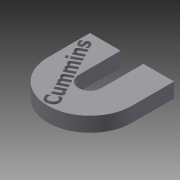
# Autodesk Inventor part: Cummins
Saved by Autodesk Inventor 2015 SP2 (Build 190223200, 223)
## iProperties
Created: 2015-09-30
Part Number: Cummins
Material: Generic
Document SubType Name: Modeling
Designer: KC-019
Density: 1 g/cm^3
Appearance: Default
Author: KC-019
Autodesk Inventor part; units mm, degrees
ref_plane "YZ Plane" through (0, 0, 0) normal (1, 0, 0) x (0, 1, 0)
ref_plane "XZ Plane" through (0, 0, 0) normal (0, 1, 0) x (-1, 0, 0)
ref_plane "XY Plane" through (0, 0, 0) normal (0, 0, 1) x (1, 0, 0)
sketch "Sketch1" plane through (0, 0, 0) normal (0, 1, 0) x (-1, 0, 0)
  line L0 (0, 0) -> (-50.8, 0)
  line L1 (-50.8, 0) -> (-50.8, -25.4)
  line L2 (-50.8, -25.4) -> (0, -25.4)
  line L3 (0, -25.4) -> (0, 0)
  arc A0 (0, 0) -> (-50.8, 0) centre (-25.4, 0) ccw
  line L4 (0, -25.4) -> (-18.5166, -25.4)
  line L5 (-18.5166, -25.4) -> (-32.2834, -25.4)
  line L6 (-32.2834, -25.4) -> (-50.8, -25.4)
  arc A1 (-18.5166, 0) -> (-32.2834, 0) centre (-25.4, 0) ccw
  line L7 (-18.5166, 0) -> (-18.5166, -25.4)
  line L8 (-32.2834, 0) -> (-32.2834, -25.4)
  dimension "d0" = 50.8
  dimension "d1" = 25.4
  dimension "d2" = 18.5166
  dimension "d3" = 13.7668
  dimension "d4" = 18.5166
  constraints: 18 end point, 4 point on circle, 4 point on line, 2 centre point, 2 parallel, 2 perpendicular, 1 coincident, 1 collinear, 1 horizontal, 1 midpoint, 1 tangent
  measures "d0" distance of L2.end L1.end
  measures "d1" distance of L0.end L1.end
  measures "d2" distance of L2.end L4.end
  measures "d3" distance of L4.end L5.end
  measures "d4" distance of L5.end L1.end
extrude "Extrusion1" add sketch "Sketch1" along normal blind 8.89 contours L3 L2 L7 L0 | L0 A1 A0 | L0 L8 L2 L1
sketch "Sketch2" plane through (0, 8.89, 0) normal (0, 1, 0) x (1, 0, 0)
  line L0 (21.5324, -26.082) -> (7.577, 0.2641)
  line L1 (7.577, 0.2641) -> (49.2759, 22.3519)
  line L2 (49.2759, 22.3519) -> (63.2313, -3.9942)
  line L3 (63.2313, -3.9942) -> (21.5324, -26.082)
  spline S0 degree 2 poles (26.8827, -18.5591) (27.6996, -20.1014) (26.7936, -22.8973) (25.1071, -23.7907) knots 0 0 0 1 2 2 2
  spline S1 degree 2 poles (25.1071, -23.7907) (23.4816, -24.6517) (20.5845, -23.8632) (19.7676, -22.3209) knots 0 0 0 1 2 2 2
  spline S2 degree 2 poles (19.7676, -22.3209) (19.553, -21.9159) (19.3006, -21.2113) (19.2196, -20.8706) knots 0 0 0 1 2 2 2
  spline S3 degree 2 poles (19.2196, -20.8706) (19.1683, -20.5994) (19.1159, -19.9238) (19.1136, -19.7048) knots 0 0 0 1 2 2 2
  line L4 (19.1136, -19.7048) -> (20.7446, -18.8409)
  line L5 (20.7446, -18.8409) -> (20.8357, -19.0128)
  spline S4 degree 2 poles (20.8357, -19.0128) (20.7923, -19.1992) (20.6815, -19.741) (20.6636, -20.056) knots 0 0 0 1 2 2 2
  spline S5 degree 2 poles (20.6636, -20.056) (20.6402, -20.3739) (20.7376, -21.054) (20.9051, -21.3702) knots 0 0 0 1 2 2 2
  spline S6 degree 2 poles (20.9051, -21.3702) (21.102, -21.7419) (21.6612, -22.2343) (22.1051, -22.3615) knots 0 0 0 1 2 2 2
  spline S7 degree 2 poles (22.1051, -22.3615) (22.501, -22.4786) (23.5675, -22.3328) (24.1722, -22.0125) knots 0 0 0 1 2 2 2
  spline S8 degree 2 poles (24.1722, -22.0125) (24.8102, -21.6745) (25.502, -20.8748) (25.6213, -20.4563) knots 0 0 0 1 2 2 2
  spline S9 degree 2 poles (25.6213, -20.4563) (25.741, -20.0519) (25.6217, -19.2768) (25.4483, -18.9495) knots 0 0 0 1 2 2 2
  spline S10 degree 2 poles (25.4483, -18.9495) (25.2691, -18.6111) (24.7154, -18.1157) (24.4651, -17.9784) knots 0 0 0 1 2 2 2
  spline S11 degree 2 poles (24.4651, -17.9784) (24.203, -17.8189) (23.7238, -17.6251) (23.5397, -17.5592) knots 0 0 0 1 2 2 2
  line L6 (23.5397, -17.5592) -> (23.4574, -17.4039)
  line L7 (23.4574, -17.4039) -> (25.0663, -16.5517)
  spline S12 degree 2 poles (25.0663, -16.5517) (25.255, -16.6933) (25.7384, -17.0695) (25.9571, -17.2946) knots 0 0 0 1 2 2 2
  spline S13 degree 2 poles (25.9571, -17.2946) (26.2274, -17.5635) (26.6241, -18.0709) (26.8827, -18.5591) knots 0 0 0 1 2 2 2
  line L8 (22.4944, -10.5966) -> (23.3466, -12.2054)
  line L9 (23.3466, -12.2054) -> (22.7752, -12.5081)
  spline S14 degree 2 poles (22.7752, -12.5081) (23.3451, -12.739) (24.0815, -13.2441) (24.3372, -13.7267) knots 0 0 0 1 2 2 2
  spline S15 degree 2 poles (24.3372, -13.7267) (24.7427, -14.4923) (24.2273, -15.8665) (23.2509, -16.3837) knots 0 0 0 1 2 2 2
  line L10 (23.2509, -16.3837) -> (19.889, -18.1645)
  line L11 (19.889, -18.1645) -> (19.0309, -16.5445)
  line L12 (19.0309, -16.5445) -> (21.594, -15.1869)
  spline S16 degree 2 poles (21.594, -15.1869) (21.9934, -14.9753) (22.4833, -14.6661) (22.6141, -14.4974) knots 0 0 0 1 2 2 2
  spline S17 degree 2 poles (22.6141, -14.4974) (22.7338, -14.3345) (22.7386, -13.9412) (22.5917, -13.6638) knots 0 0 0 1 2 2 2
  spline S18 degree 2 poles (22.5917, -13.6638) (22.5036, -13.4974) (22.0903, -13.1195) (21.8432, -13.0018) knots 0 0 0 1 2 2 2
  line L13 (21.8432, -13.0018) -> (18.1817, -14.9412)
  line L14 (18.1817, -14.9412) -> (17.3295, -13.3324)
  line L15 (17.3295, -13.3324) -> (22.4944, -10.5966)
  line L16 (18.5773, -3.2014) -> (15.9976, -4.5679)
  spline S19 degree 2 poles (15.9976, -4.5679) (15.6148, -4.7706) (15.108, -5.0746) (14.9768, -5.2293) knots 0 0 0 1 2 2 2
  spline S20 degree 2 poles (14.9768, -5.2293) (14.8486, -5.3896) (14.8516, -5.7574) (14.9897, -6.0182) knots 0 0 0 1 2 2 2
  spline S21 degree 2 poles (14.9897, -6.0182) (15.0867, -6.2013) (15.4356, -6.4711) (15.6971, -6.6026) knots 0 0 0 1 2 2 2
  line L17 (15.6971, -6.6026) -> (19.353, -4.666)
  line L18 (19.353, -4.666) -> (20.2111, -6.286)
  line L19 (20.2111, -6.286) -> (17.6314, -7.6524)
  spline S22 degree 2 poles (17.6314, -7.6524) (17.2542, -7.8522) (16.7448, -8.1647) (16.6136, -8.3194) knots 0 0 0 1 2 2 2
  spline S23 degree 2 poles (16.6136, -8.3194) (16.4854, -8.4797) (16.4884, -8.8475) (16.6265, -9.1083) knots 0 0 0 1 2 2 2
  spline S24 degree 2 poles (16.6265, -9.1083) (16.7294, -9.3024) (17.1152, -9.5883) (17.3368, -9.6982) knots 0 0 0 1 2 2 2
  line L20 (17.3368, -9.6982) -> (20.9928, -7.7617)
  line L21 (20.9928, -7.7617) -> (21.845, -9.3705)
  line L22 (21.845, -9.3705) -> (16.6801, -12.1063)
  line L23 (16.6801, -12.1063) -> (15.8279, -10.4975)
  line L24 (15.8279, -10.4975) -> (16.3993, -10.1948)
  spline S25 degree 2 poles (16.3993, -10.1948) (15.8578, -9.9773) (15.1073, -9.4725) (14.8752, -9.0343) knots 0 0 0 1 2 2 2
  spline S26 degree 2 poles (14.8752, -9.0343) (14.6254, -8.5627) (14.6927, -7.6035) (15.0422, -7.1768) knots 0 0 0 1 2 2 2
  spline S27 degree 2 poles (15.0422, -7.1768) (14.3656, -6.9456) (13.4646, -6.3713) (13.2413, -5.9497) knots 0 0 0 1 2 2 2
  spline S28 degree 2 poles (13.2413, -5.9497) (13.0503, -5.5891) (12.9751, -4.8972) (13.1052, -4.5796) knots 0 0 0 1 2 2 2
  spline S29 degree 2 poles (13.1052, -4.5796) (13.2403, -4.231) (13.808, -3.6532) (14.3573, -3.3623) knots 0 0 0 1 2 2 2
  line L25 (14.3573, -3.3623) -> (17.7192, -1.5815)
  line L26 (17.7192, -1.5815) -> (18.5773, -3.2014)
  line L27 (13.8226, 5.7748) -> (11.2429, 4.4083)
  spline S30 degree 2 poles (11.2429, 4.4083) (10.8601, 4.2056) (10.3533, 3.9016) (10.2221, 3.7469) knots 0 0 0 1 2 2 2
  spline S31 degree 2 poles (10.2221, 3.7469) (10.0939, 3.5866) (10.0969, 3.2188) (10.235, 2.958) knots 0 0 0 1 2 2 2
  spline S32 degree 2 poles (10.235, 2.958) (10.332, 2.775) (10.681, 2.5051) (10.9424, 2.3737) knots 0 0 0 1 2 2 2
  line L28 (10.9424, 2.3737) -> (14.5984, 4.3102)
  line L29 (14.5984, 4.3102) -> (15.4564, 2.6903)
  line L30 (15.4564, 2.6903) -> (12.8768, 1.3238)
  spline S33 degree 2 poles (12.8768, 1.3238) (12.4995, 1.124) (11.9901, 0.8115) (11.8589, 0.6568) knots 0 0 0 1 2 2 2
  spline S34 degree 2 poles (11.8589, 0.6568) (11.7307, 0.4965) (11.7337, 0.1287) (11.8718, -0.132) knots 0 0 0 1 2 2 2
  spline S35 degree 2 poles (11.8718, -0.132) (11.9747, -0.3262) (12.3605, -0.612) (12.5822, -0.722) knots 0 0 0 1 2 2 2
  line L31 (12.5822, -0.722) -> (16.2381, 1.2146)
  line L32 (16.2381, 1.2146) -> (17.0903, -0.3943)
  line L33 (17.0903, -0.3943) -> (11.9254, -3.1301)
  line L34 (11.9254, -3.1301) -> (11.0732, -1.5213)
  line L35 (11.0732, -1.5213) -> (11.6446, -1.2186)
  spline S36 degree 2 poles (11.6446, -1.2186) (11.1031, -1.001) (10.3526, -0.4963) (10.1205, -0.058) knots 0 0 0 1 2 2 2
  spline S37 degree 2 poles (10.1205, -0.058) (9.8707, 0.4135) (9.9381, 1.3728) (10.2875, 1.7994) knots 0 0 0 1 2 2 2
  spline S38 degree 2 poles (10.2875, 1.7994) (9.6109, 2.0307) (8.71, 2.6049) (8.4866, 3.0265) knots 0 0 0 1 2 2 2
  spline S39 degree 2 poles (8.4866, 3.0265) (8.2956, 3.3871) (8.2204, 4.079) (8.3505, 4.3966) knots 0 0 0 1 2 2 2
  spline S40 degree 2 poles (8.3505, 4.3966) (8.4856, 4.7452) (9.0534, 5.323) (9.6026, 5.6139) knots 0 0 0 1 2 2 2
  line L36 (9.6026, 5.6139) -> (12.9645, 7.3947)
  line L37 (12.9645, 7.3947) -> (13.8226, 5.7748)
  line L38 (11.4805, 10.1963) -> (12.3327, 8.5875)
  line L39 (12.3327, 8.5875) -> (7.1678, 5.8517)
  line L40 (7.1678, 5.8517) -> (6.3156, 7.4605)
  line L41 (6.3156, 7.4605) -> (11.4805, 10.1963)
  line L42 (5.5513, 7.1196) -> (6.4534, 5.4164)
  line L43 (6.4534, 5.4164) -> (5.1996, 4.7523)
  line L44 (5.1996, 4.7523) -> (4.2975, 6.4555)
  line L45 (4.2975, 6.4555) -> (5.5513, 7.1196)
  line L46 (8.2686, 16.26) -> (9.1267, 14.6401)
  line L47 (9.1267, 14.6401) -> (6.5692, 13.2854)
  spline S41 degree 2 poles (6.5692, 13.2854) (6.253, 13.1179) (5.6581, 12.7388) (5.5491, 12.5958) knots 0 0 0 1 2 2 2
  spline S42 degree 2 poles (5.5491, 12.5958) (5.4156, 12.4186) (5.4304, 12.0286) (5.5715, 11.7623) knots 0 0 0 1 2 2 2
  spline S43 degree 2 poles (5.5715, 11.7623) (5.6743, 11.5681) (6.0386, 11.2425) (6.32, 11.1002) knots 0 0 0 1 2 2 2
  line L48 (6.32, 11.1002) -> (9.9759, 13.0368)
  line L49 (9.9759, 13.0368) -> (10.8281, 11.4279)
  line L50 (10.8281, 11.4279) -> (5.6632, 8.6921)
  line L51 (5.6632, 8.6921) -> (4.811, 10.3009)
  line L52 (4.811, 10.3009) -> (5.3824, 10.6036)
  spline S44 degree 2 poles (5.3824, 10.6036) (4.8409, 10.8212) (4.067, 11.3703) (3.826, 11.8252) knots 0 0 0 1 2 2 2
  spline S45 degree 2 poles (3.826, 11.8252) (3.4087, 12.613) (3.9636, 13.9796) (4.9067, 14.4792) knots 0 0 0 1 2 2 2
  line L53 (4.9067, 14.4792) -> (8.2686, 16.26)
  spline S46 degree 2 poles (6.9439, 19.0962) (7.2436, 18.5304) (7.5317, 17.3829) (7.5416, 16.9619) knots 0 0 0 1 2 2 2
  line L54 (7.5416, 16.9619) -> (6.1824, 16.2419)
  line L55 (6.1824, 16.2419) -> (6.1119, 16.3751)
  spline S47 degree 2 poles (6.1119, 16.3751) (6.1389, 16.5386) (6.194, 16.9443) (6.1724, 17.2667) knots 0 0 0 1 2 2 2
  spline S48 degree 2 poles (6.1724, 17.2667) (6.1573, 17.55) (6.0103, 18.1897) (5.834, 18.5226) knots 0 0 0 1 2 2 2
  spline S49 degree 2 poles (5.834, 18.5226) (5.6547, 18.861) (5.1677, 19.2708) (4.9402, 19.1503) knots 0 0 0 1 2 2 2
  spline S50 degree 2 poles (4.9402, 19.1503) (4.7627, 19.0563) (4.7004, 18.7178) (4.805, 18.3327) knots 0 0 0 1 2 2 2
  spline S51 degree 2 poles (4.805, 18.3327) (4.852, 18.1232) (5.0434, 17.507) (5.0914, 17.2554) knots 0 0 0 1 2 2 2
  spline S52 degree 2 poles (5.0914, 17.2554) (5.2261, 16.5452) (4.8115, 15.5442) (4.2068, 15.2238) knots 0 0 0 1 2 2 2
  spline S53 degree 2 poles (4.2068, 15.2238) (3.8628, 15.0417) (3.0851, 15.0346) (2.6819, 15.2189) knots 0 0 0 1 2 2 2
  spline S54 degree 2 poles (2.6819, 15.2189) (2.2873, 15.4006) (1.5309, 16.158) (1.2283, 16.7294) knots 0 0 0 1 2 2 2
  spline S55 degree 2 poles (1.2283, 16.7294) (0.9403, 17.2731) (0.6747, 18.2975) (0.6599, 18.6875) knots 0 0 0 1 2 2 2
  line L56 (0.6599, 18.6875) -> (1.9692, 19.381)
  line L57 (1.9692, 19.381) -> (2.0368, 19.2534)
  spline S56 degree 2 poles (2.0368, 19.2534) (2.0143, 19.135) (1.9889, 18.6598) (1.9994, 18.4522) knots 0 0 0 1 2 2 2
  spline S57 degree 2 poles (1.9994, 18.4522) (2.0194, 18.1999) (2.1618, 17.636) (2.2999, 17.3752) knots 0 0 0 1 2 2 2
  spline S58 degree 2 poles (2.2999, 17.3752) (2.4851, 17.0257) (2.9793, 16.6694) (3.1734, 16.7723) knots 0 0 0 1 2 2 2
  spline S59 degree 2 poles (3.1734, 16.7723) (3.351, 16.8663) (3.4243, 17.2106) (3.3126, 17.663) knots 0 0 0 1 2 2 2
  spline S60 degree 2 poles (3.3126, 17.663) (3.2538, 17.8947) (3.0631, 18.4828) (3.0141, 18.7765) knots 0 0 0 1 2 2 2
  spline S61 degree 2 poles (3.0141, 18.7765) (2.8977, 19.4253) (3.2856, 20.3696) (3.8625, 20.6752) knots 0 0 0 1 2 2 2
  spline S62 degree 2 poles (3.8625, 20.6752) (4.2231, 20.8662) (5.0626, 20.8775) (5.452, 20.6788) knots 0 0 0 1 2 2 2
  spline S63 degree 2 poles (5.452, 20.6788) (5.8695, 20.4808) (6.6118, 19.7231) (6.9439, 19.0962) knots 0 0 0 1 2 2 2
  point P0 (0, 0)
  constraints: 2 other
extrude "Extrusion2" cut sketch "Sketch2" against normal through all contours S37 S38 S39 S40 L36 L37 L27 S30 S31 S32 L28 L29 L1 | L1 L29 L30 S33 S34 S35 L31 L32 L33 L34 L35 S36 S37 | S0 S1 S2 S3 L4 L5 S4 S5 S6 S7 S8 S9 S10 S11 L6 L7 S12 S13 | L8 L9 S14 S15 L10 L11 L12 S16 S17 S18 L13 L14 L15 | L16 S19 S20 S21 L17 L18 L19 S22 S23 S24 L20 L21 L22 L23 L24 S25 S26 S27 S28 S29 L25 L26 | L38 L39 L40 L41 | L42 L43 L44 L45 | L46 L47 S41 S42 S43 L48 L49 L50 L51 L52 S44 S45 L53 | S46 L54 L55 S47 S48 S49 S50 S51 S52 S53 S54 S55 L56 L57 S56 S57 S58 S59 S60 S61 S62 S63
body "Solid1"
